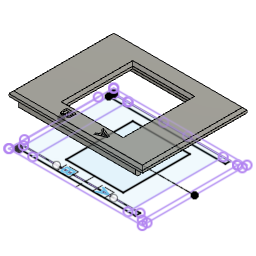
vga-adapter-fusion360 (Autodesk Fusion 360 design; units mm, degrees)
Autodesk Fusion 360 part; units mm, degrees
sketch "Sketch1" plane through (0, 0, 0) normal (0, 0, 1) x (1, 0, 0)
  line L0 (0, 0) -> (52, 0)
  line L1 (52, 0) -> (52, 40)
  line L2 (52, 40) -> (0, 40)
  line L3 (0, 40) -> (0, 0)
  line L4 (54, -2) -> (54, 42)
  line L5 (54, 42) -> (-2, 42)
  line L6 (-2, 42) -> (-2, -2)
  line L7 (-2, -2) -> (54, -2)
  line L8 (-2, 20) -> (0, 20) construction
  line L9 (-2, 35.5) -> (0, 35.5)
  line L10 (0, 35.5) -> (0, 4.5)
  line L11 (0, 4.5) -> (-2, 4.5)
  line L12 (-2, 4.5) -> (-2, 35.5)
  line L13 (52, 40) -> (54, 40)
  line L14 (54, 40) -> (54, 0)
  line L15 (54, 0) -> (52, 0)
  line L16 (52, 0) -> (52, 40)
  line L17 (0, 0) -> (6, 0)
  line L18 (6, 0) -> (6, 40)
  line L19 (6, 40) -> (0, 40)
  line L20 (0, 40) -> (0, 0)
  line L21 (52, 0) -> (46, 0)
  line L22 (46, 0) -> (46, 40)
  line L23 (46, 40) -> (52, 40)
  line L24 (52, 40) -> (52, 0)
  line L25 (31, 0) -> (21, 0)
  line L26 (21, 0) -> (21, 40)
  line L27 (21, 40) -> (31, 40)
  line L28 (31, 40) -> (31, 0)
  line L29 (0, 0) -> (0, 4.5)
  line L30 (-2, 20) -> (54, 20) construction
  dimension "d1" = 40
  dimension "d2" = 52
  dimension "d3" = 2
  dimension "d4" = 31
  dimension "d11" = 6
  dimension "d12" = 6
  dimension "d13" = 10
  constraint horizontal L0
  constraint vertical L1
  constraint horizontal L2
  constraint vertical L3
  constraint coincident L0.start L3.end
  constraint midpoint L6 L8.start
  constraint midpoint L3 L8.end
  constraint horizontal L9
  constraint vertical L10
  constraint horizontal L11
  constraint vertical L12
  constraint coincident L3 L10.end
  constraint coincident L6 L9.start
  constraint midpoint L8.end L10
  constraint horizontal L13
  constraint vertical L14
  constraint horizontal L15
  constraint vertical L16
  constraint coincident L4 L14.end
  constraint coincident L0.end L15
  constraint horizontal L17
  constraint vertical L18
  constraint horizontal L19
  constraint vertical L20
  constraint coincident L2 L18.end
  constraint horizontal L21
  constraint vertical L22
  constraint horizontal L23
  constraint vertical L24
  constraint coincident L2 L22.end
  constraint horizontal L25
  constraint vertical L26
  constraint horizontal L27
  constraint vertical L28
  constraint coincident L2 L26.end
  constraint coincident L0 L25.start
  constraint midpoint L0 L25
  constraint vertical L29
  constraint midpoint L14 L30.end
  measures "d1" distance of L0.end L1.end
  measures "d2" distance of L1.end L2.end
  measures "d4" distance of L9 L11
  measures "d11" distance of L10 L18
  measures "d12" distance of L22 L24
  measures "d13" distance of L26 L28
extrude "Extrude1" add sketch "Sketch1" along normal blind 2 contours L0 L2 L3 L10 L17 L18 L19 L20 L29 | L0 L2 L18 L26 | L0 L2 L25 L26 L27 L28 | L0 L2 L22 L28 | L0 L1 L2 L16 L21 L22 L23 L24 makes body 1
extrude "Extrude2" add sketch "Sketch1" along normal blind 19 contours L0 L3 L4 L6 L7 L11 L15 L17 L20 L21 L25 L29 | L2 L3 L4 L5 L6 L9 L13 L19 L20 L23 L27 bodies 1
extrude "Extrude3" add sketch "Sketch1" along normal blind 6 contours L3 L6 L9 L10 L11 L12 L20 | L1 L4 L13 L14 L15 L16 L24 bodies 1
extrude "Extrude5" add sketch "Sketch1" along normal blind 4 contours L0 L2 L25 L26 L27 L28 | L0 L1 L2 L16 L21 L22 L23 L24 bodies 1
extrude "Extrude6" add sketch "Sketch1" along normal blind 6 contours L0 L2 L3 L10 L17 L18 L19 L20 L29 bodies 1
chamfer "Chamfer2" distance 1 angle 45 4 edges at (26, 42, 0) (54, 20, 0) (-2, 20, 0) (26, -2, 0) on bodies 1
extrude "Extrude1'" add sketch "Sketch1" along normal blind 2 from surface at 19 separate body makes body 2 in component "Component"
sketch "Sketch1 (2)" plane through (0, 0, 0) normal (0, 0, 1) x (1, 0, 0) in component "Component"
  line L0 (49, 39.9) -> (0, 39.9)
  line L1 (0, 37.9) -> (49, 37.9)
  line L2 (49, 37.9) -> (49, 39.9)
  line L3 (52, 20) -> (0, 20) construction
  line L4 (0, 40) -> (0, 0)
  line L5 (52, 0) -> (52, 40)
  line L6 (6, 40) -> (0, 40)
  line L7 (6, 0) -> (6, 40)
  line L8 (46, 0) -> (46, 40)
  line L9 (52, 40) -> (0, 40)
  line L10 (21, 40) -> (31, 40)
  line L11 (0, 37.9) -> (0, 40)
  line L12 (0, 2.1) -> (0, 0)
  line L13 (0, 2.1) -> (49, 2.1)
  line L14 (49, 0.1) -> (0, 0.1)
  line L15 (49, 2.1) -> (49, 0.1)
  dimension "d25" = 2
  dimension "d26" = 0.1
  dimension "d38" = 3
  constraint horizontal L0
  constraint horizontal L1
  constraint vertical L2
  constraint horizontal L3
  constraint midpoint L3.end L4
  constraint midpoint L3.start L5
  constraint coincident L4 L1.start
  constraint coincident L4.start L6.end
  constraint symmetric L0.start L3 L14.start
  constraint symmetric L1.end L3 L13.end
  constraint symmetric L3 L0.end L14.end
  constraint symmetric L3 L1.start L12.start
  constraint symmetric L3 L4.start L4.end
  measures "d25" distance of L0 L1
  measures "d26" distance of L0 L10
  measures "d38" distance of L2 L5
extrude "Extrude2'" add sketch "Sketch1 (2)" against normal blind 5 from surface at 19 contours L0 L1 L2 L8 | L0 L1 L7 L8 | L0 L1 L4 L7 L11 | L8 L13 L14 L15 | L7 L8 L13 L14 | L4 L7 L12 L13 L14 bodies 2 in component "Component"
sketch "Sketch2" plane through (0, 0, 0) normal (0, 0, 1) x (1, 0, 0) in component "Component"
  line L0 (38, 6) -> (14, 6)
  line L1 (14, 6) -> (14, 34)
  line L2 (14, 34) -> (38, 34)
  line L3 (38, 34) -> (38, 6)
  line L4 (-2, 4.5) -> (-2, 35.5)
  line L5 (54, 40) -> (54, 0)
  line L6 (-2, -2) -> (54, -2)
  line L7 (54, 20) -> (-2, 20) construction
  line L8 (-2, 42) -> (-2, -2)
  line L9 (54, 42) -> (-2, 42)
  line L10 (26, 6) -> (26, -2) construction
  line L11 (14, 2) -> (38, 2) construction
  line L12 (31, 4.1) -> (31, 0.1) construction
  line L13 (31, 0.1) -> (36, 0.1) construction
  line L14 (36, 0.1) -> (36, 4.1) construction
  line L15 (36, 4.1) -> (31, 4.1) construction
  line L16 (0, 2.1) -> (49, 2.1) construction
  line L17 (16, 4.1) -> (16, 0.1) construction
  line L18 (16, 0.1) -> (21, 0.1) construction
  line L19 (21, 0.1) -> (21, 4.1) construction
  line L20 (21, 4.1) -> (16, 4.1) construction
  dimension "d27" = 16
  dimension "d28" = 16
  dimension "d29" = 8
  dimension "d30" = 8
  dimension "d49" = 4
  dimension "d50" = 4
  dimension "d51" = 5
  dimension "d52" = 4
  dimension "d53" = 4
  dimension "d54" = 5
  dimension "d55" = 10
  text T0 "A" font "Arial" height 4 bold align centre middle in box 4 x 5 at (31, 4.1) x (0, -1) y (1, 0) spacing 1 kerned
  text T1 "B" font "Arial" height 4 bold align centre middle in box 4 x 5 at (16, 4.1) x (0, -1) y (1, 0) spacing 1 kerned
  constraint horizontal L0
  constraint vertical L1
  constraint horizontal L2
  constraint vertical L3
  constraint coincident L5 L7.start
  constraint coincident L4 L7.end
  constraint perpendicular L4 L7
  constraint midpoint L7.end L8
  constraint midpoint L0 L10.start
  constraint midpoint L6 L10.end
  constraint horizontal L11
  constraint midpoint L10 L11
  measures "d27" distance of L1 L4
  measures "d28" distance of L3 L5
  measures "d29" distance of L0 L6
  measures "d30" distance of L2 L9
  measures "d50" distance of L13 L15
  measures "d51" distance of L12 L14
  measures "d53" distance of L18 L20
  measures "d54" distance of L17 L19
  measures "d55" distance of L12 L19
extrude "Extrude3'" cut sketch "Sketch2" along normal through all from surface at 19 bodies 2 in component "Component"
chamfer "Chamfer3" distance 1 angle 45 10 edges at (26, -2, 21) (-2, 20, 21) (54, 20, 21) (26, 42, 21) (38, 20, 21) (26, 34, 21) (26, 6, 21) (14, 20, 21) (24.5, 39.9, 14) (24.5, 0.1, 14) on bodies 2 in component "Component"
extrude "Extrude4" cut sketch "Sketch2" against normal blind 1 from surface at 21 text T1 T0 bodies 2 in component "Component"
component "Component" placed x (1, 0, 0) y (0, 1, 0) z (0, 0, 1) at (0, 0, 0)
equation "d30 = d29"
